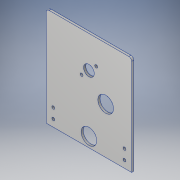
# Autodesk Inventor part: 板3
Saved by Autodesk Inventor 2019 (Build 230136000, 136)
## iProperties
Created: 2020-09-28
Part Number: 板3
Material: アルミニウム 6061
Document SubType Name: Modeling
Designer: zhept
Density: 2.7 g/cm^3
Appearance: アルミニウム - フラット
Mass: 128.079 g
Surface Area: 338.754 cm^2
Volume: 47.4367 cm^3
Author: zhept
Autodesk Inventor part; units mm, degrees
ref_plane "YZ Plane" through (0, 0, 0) normal (1, 0, 0) x (0, 1, 0)
ref_plane "XZ Plane" through (0, 0, 0) normal (0, 1, 0) x (-1, 0, 0)
ref_plane "XY Plane" through (0, 0, 0) normal (0, 0, 1) x (1, 0, 0)
sketch "スケッチ1" plane through (0, 0, 0) normal (0, 0, 1) x (1, 0, 0)
  circle A0 centre (0, 0) radius 7.5
  circle A1 centre (0, 0) radius 30
  circle A2 centre (0, 0) radius 37.5
  circle A3 centre (23.5425, -29.1891) radius 30
  circle A4 centre (23.5425, -29.1891) radius 4
  circle A5 centre (23.5425, -29.1891) radius 16
  circle A6 centre (23.5425, -29.1891) radius 56
  circle A7 centre (0, -80) radius 40
  circle A8 centre (0, -80) radius 50
  circle A9 centre (0, -80) radius 4
  dimension "d57" = 75
  dimension "d64" = 112
  dimension "d41" = 15
  dimension "d58" = 8
  dimension "d63" = 32
  dimension "d65" = 100
  dimension "d66" = 8
  constraints: 9 coincident, 8 centre point, 2 tangent, 6 other
  measures "d41" diameter of A0
  measures "d58" diameter of A4
  measures "d63" diameter of A5
  measures "d65" diameter of A8
  measures "d66" diameter of A9
sketch "スケッチ2" plane through (0, 0, 0) normal (0, 0, 1) x (1, 0, 0)
  line L0 (0, 0) -> (24.502, 0) construction
  line L1 (0, 0) -> (12.5, 0) construction
  line L2 (0, 0) -> (10.253, 10.253)
  line L3 (0, 0) -> (14.5, 0) construction
  line L4 (10.253, 10.253) -> (-10.253, -10.253)
  circle A0 centre (10.253, 10.253) radius 2
  circle A1 centre (-10.253, -10.253) radius 2
  circle A2 centre (0, 0) radius 7.5
  line L5 (0, 0) -> (28.1908, 10.2606)
  line L6 (0, 0) -> (30, 0) construction
  line L7 (0, 0) -> (-28.1908, 10.2606)
  line L8 (0, 0) -> (30, 0) construction
  circle A3 centre (-28.1908, 10.2606) radius 2.5
  line L9 (0, 0) -> (0, 30)
  circle A4 centre (0, 30) radius 2.5
  circle A5 centre (28.1908, 10.2606) radius 2.5
  dimension "d9" = 14.5
  dimension "d10" = 45
  dimension "d11" = 29
  dimension "d12" = 4
  dimension "d13" = 4
  dimension "d14" = 15
  dimension "d15" = 30
  dimension "d16" = 20
  dimension "d17" = 30
  dimension "d18" = 160
  dimension "d19" = 5
  dimension "d20" = 30
  dimension "d21" = 5
  dimension "d22" = 5
  constraints: 20 end point, 6 centre point, 6 coincident, 5 horizontal, 3 equal length, 1 point on line, 1 vertical
  measures "d9" distance of L0.start L2.end
  measures "d10" angle of L3 L2
  measures "d11" distance of L2.end L4.end
  measures "d12" diameter of A0
  measures "d13" diameter of A1
  measures "d14" diameter of A2
  measures "d15" distance of L5.start L5.end
  measures "d16" angle of L6 L5
  measures "d17" distance of L5.start L7.end
  measures "d18" angle of L8 L7
  measures "d19" diameter of A3
  measures "d20" distance of L5.start L9.end
  measures "d21" diameter of A4
  measures "d22" diameter of A5
sketch "スケッチ3" plane through (0, 0, 0) normal (0, 0, 1) x (1, 0, 0)
  line L0 (60, -99.3436) -> (-60, -99.3436)
  line L1 (-60, -99.3436) -> (-60, 99.3436)
  line L2 (-60, 99.3436) -> (60, 99.3436)
  line L3 (60, 99.3436) -> (60, -99.3436)
  line L4 (60, -99.3436) -> (-60, 99.3436) construction
  line L5 (-60, -99.3436) -> (60, 99.3436) construction
  point P0 (0, 0)
  dimension "d25" = 120
  constraints: 12 end point, 2 midpoint, 2 parallel, 1 horizontal, 1 perpendicular
  measures "d25" distance of L0.start L0.end
extrude "押し出し1" add sketch "スケッチ3" against normal blind 3
sketch "スケッチ4" plane through (0, 0, 0) normal (0, 0, 1) x (1, 0, 0)
  line L0 (0, 45.0711) -> (68.3595, 45.0711)
  line L1 (68.3595, 45.0711) -> (-74.3824, 45.0711)
  line L2 (-74.3824, 45.0711) -> (108.1656, 45.0711)
  line L3 (108.1656, 45.0711) -> (108.1656, 129.4154)
  line L4 (108.1656, 129.4154) -> (-74.3824, 129.4154)
  line L5 (-74.3824, 129.4154) -> (-74.3824, 45.0711)
  point P0 (0, 0)
  constraints: 12 end point, 2 horizontal, 2 parallel, 1 perpendicular, 1 point on line
extrude "押し出し4" cut sketch "スケッチ4" against normal blind 10
fillet "フィレット1" radius 4 4 edges at (-60, 45.0711, -1.5) (60, 45.0711, -1.5) (-60, -99.3436, -1.5) (60, -99.3436, -1.5)
extrude "押し出し9" cut sketch "スケッチ1" against normal blind 10 contours A4 A2 | A2 A4 | A9 A6 | A6 A9
sketch "スケッチ8" plane through (0, 0, 0) normal (0, 0, 1) x (1, 0, 0)
  line L0 (-265.6992, -158.784) -> (100.3409, -158.784)
  line L1 (100.3409, -158.784) -> (100.3409, -94)
  line L2 (100.3409, -94) -> (-265.6992, -94)
  line L3 (-265.6992, -94) -> (-265.6992, -158.784)
  line L4 (-265.6992, -158.784) -> (100.3409, -94) construction
  line L5 (100.3409, -158.784) -> (-265.6992, -94) construction
  point P0 (0, 0)
  point P1 (0, -94)
  point P2 (-82.6791, -126.392)
  constraints: 12 end point, 2 midpoint, 2 parallel, 1 horizontal, 1 perpendicular
extrude "押し出し10" cut sketch "スケッチ8" against normal blind 10
sketch "スケッチ9" plane through (0, 0, 0) normal (0, 0, 1) x (1, 0, 0)
  circle A0 centre (-50, -84) radius 2
  circle A1 centre (50, -84) radius 2
  circle A2 centre (-50, -70) radius 2
  circle A3 centre (50, -70) radius 2
  point P0 (0, 0)
  dimension "d73" = 4
  dimension "d74" = 4
  dimension "d75" = 4
  dimension "d76" = 4
  constraints: 4 centre point
  measures "d73" diameter of A0
  measures "d74" diameter of A1
  measures "d75" diameter of A2
  measures "d76" diameter of A3
extrude "押し出し12" cut sketch "スケッチ9" against normal blind 10
sketch "スケッチ10" plane through (0, 0, -3) normal (0, 0, -1) x (-1, 0, 0)
  circle A0 centre (-23.5425, -29.1891) radius 4 projected
  circle A1 centre (-23.5425, -29.1891) radius 11
  circle A2 centre (0, -80) radius 4 projected
  circle A3 centre (0, -80) radius 11
  point P0 (0, 0)
  dimension "d79" = 22
  dimension "d80" = 22
  constraints: 2 centre point, 2 coincident
  measures "d79" diameter of A1
  measures "d80" diameter of A3
extrude "押し出し13" cut sketch "スケッチ10" against normal blind 10
extrude "押し出し14" cut sketch "スケッチ2" against normal blind 10 contours L9 A2 L2 | L5 A2 L4 | L2 A2 L5 | L4 A2 L7 | L7 A2 L9 | A0 | A1
